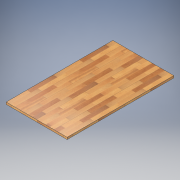
# Autodesk Inventor part: tabletop
Saved by Autodesk Inventor 2019 (Build 230136000, 136)
## iProperties
Created: 2019-04-29
Part Number: tabletop
Material: Wood Flooring
Document SubType Name: Modeling
Designer: Alex
Density: 0.673 g/cm^3
Appearance: Beechwood - Galliano
Author: Alex
Autodesk Inventor part; units mm, degrees
ref_plane "YZ Plane" through (0, 0, 0) normal (1, 0, 0) x (0, 1, 0)
ref_plane "XZ Plane" through (0, 0, 0) normal (0, 1, 0) x (-1, 0, 0)
ref_plane "XY Plane" through (0, 0, 0) normal (0, 0, 1) x (1, 0, 0)
sketch "Sketch1" plane through (0, 0, 0) normal (0, 1, 0) x (-1, 0, 0)
  line L0 (364.3564, 546.5346) -> (-435.6436, 546.5346)
  line L1 (-435.6436, 546.5346) -> (-435.6436, -853.4654)
  line L2 (-435.6436, -853.4654) -> (364.3564, -853.4654)
  line L3 (364.3564, -853.4654) -> (364.3564, 546.5346)
  point P0 (0, 0)
  dimension "d0" = 800
  dimension "d1" = 1400
  constraints: 8 end point, 2 parallel, 1 horizontal, 1 perpendicular
  measures "d0" distance of L0.start L0.end
  measures "d1" distance between parallel lines of L2 L0
extrude "Extrusion1" add sketch "Sketch1" along normal blind 27
body "Solid1"
